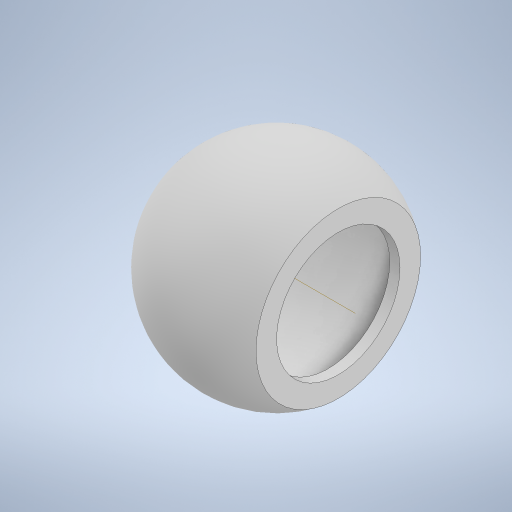
# Autodesk Inventor part: IndicatorLampCover
Saved by Autodesk Inventor 2024.2 (Build 282272000, 272)
## iProperties
Created: 2024-04-04
Part Number: IndicatorLampCover
Material: Generic
Document SubType Name: Modeling
Designer: ringl
Density: 1 g/cm^3
Appearance: Default
Author: ringl
Autodesk Inventor part; units mm, degrees
ref_plane "YZ Plane" through (0, 0, 0) normal (1, 0, 0) x (0, 1, 0)
ref_plane "XZ Plane" through (0, 0, 0) normal (0, 1, 0) x (-1, 0, 0)
ref_plane "XY Plane" through (0, 0, 0) normal (0, 0, 1) x (1, 0, 0)
sketch "Sketch1" plane through (0, 0, 0) normal (0, 1, 0) x (-1, 0, 0)
  arc A0 (0, -4) -> (8, 0) centre (3, 0) ccw
  arc A1 (0.5, -3.8) -> (7.5486, 0) centre (3, 0) ccw
  line L0 (0, -4) -> (0, -3)
  line L1 (0, -3) -> (0.5, -3)
  line L2 (0.5, -3) -> (0.5, -3.8)
  line L3 (8, 0) -> (7.5486, 0)
  line L4 (11.0833, 0) -> (-1.8472, 0) projected
  point P0 (0, 0)
  point P1 (0, 0)
  dimension "d1" = 10
  dimension "d5" = 4
  dimension "d6" = 1
  dimension "d7" = 0.5
  dimension "d8" = 0.8
  dimension "d9" = 8
  dimension "d10" = 0.4514
  constraints: 8 end point, 4 point on circle, 2 centre point, 2 coincident, 1 horizontal, 1 horizontal alignment, 1 perpendicular, 1 vertical, 1 vertical alignment
  measures "d1" diameter of A0
  measures "d5" distance of L0.start point (0, 0)
  measures "d6" distance of L0.start L0.end
  measures "d7" distance of L0.end L1.end
  measures "d8" distance of L2.end L1.end
  measures "d9" distance of point (0, 0) L3.start
  measures "d10" distance of L3.start L3.end
revolve "Revolution1" add sketch "Sketch1" angle 360 about axis through (-10, 0, 0) along (1, 0, 0)
body "Solid1"
